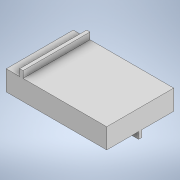
# Autodesk Inventor part: 水平滑盖
Saved by Autodesk Inventor 2020 (Build 240168000, 168)
## iProperties
Created: 2021-04-06
Part Number: 水平滑盖
Material: 常规
Document SubType Name: Modeling
Designer: 70929
Density: 1 g/cm^3
Appearance: 默认
Author: 70929
Autodesk Inventor part; units mm, degrees
ref_plane "YZ Plane" through (0, 0, 0) normal (1, 0, 0) x (0, 1, 0)
ref_plane "XZ Plane" through (0, 0, 0) normal (0, 1, 0) x (-1, 0, 0)
ref_plane "XY Plane" through (0, 0, 0) normal (0, 0, 1) x (1, 0, 0)
sketch "草图3" plane through (0, 0, 0) normal (0, 1, 0) x (-1, 0, 0)
  line L0 (-75, 50) -> (75, 50)
  line L1 (75, 50) -> (75, -50)
  line L2 (75, -50) -> (-75, -50)
  line L3 (-75, -50) -> (-75, 50)
  line L4 (-75, 50) -> (75, -50) construction
  line L5 (75, 50) -> (-75, -50) construction
  point P0 (0, 0)
  dimension "d21" = 150
  dimension "d22" = 100
  constraints: 12 end point, 2 midpoint, 2 parallel, 1 horizontal, 1 perpendicular
  measures "d21" distance of L1.end L2.end
  measures "d22" distance of L2.end L0.start
extrude "拉伸3" add sketch "草图3" against normal mid plane 30
sketch "草图4" plane through (0, 15, 0) normal (0, 1, 0) x (1, 0, 0)
  line L0 (-75, -50) -> (-55, -50)
  line L1 (75, -50) -> (-75, -50) projected
  line L2 (-55, -50) -> (-55, 50)
  line L3 (-55, 50) -> (-50, 50)
  line L4 (-75, 50) -> (75, 50) projected
  line L5 (-50, 50) -> (-50, -50)
  line L6 (-50, -50) -> (-55, -50)
  point P0 (0, 0)
  dimension "d25" = 20
  dimension "d31" = 5
  constraints: 10 end point, 3 perpendicular, 3 point on line
  measures "d25" distance of L0.start L0.end
  measures "d31" distance of L2.end L3.end
extrude "拉伸4" add sketch "草图4" along normal blind 10
sketch "草图5" plane through (0, -15, 0) normal (0, -1, 0) x (1, 0, 0)
  line L0 (75, 50) -> (75, -50) projected
  line L1 (-75, 2.5) -> (75, 2.5)
  line L2 (75, 2.5) -> (75, -2.5)
  line L3 (75, -2.5) -> (-75, -2.5)
  line L4 (-75, -2.5) -> (-75, 2.5)
  line L5 (-75, 2.5) -> (75, -2.5) construction
  line L6 (75, 2.5) -> (-75, -2.5) construction
  point P0 (0, 0)
  point P1 (75, 2.5)
  dimension "d28" = 5
  constraints: 12 end point, 2 midpoint, 2 parallel, 1 horizontal, 1 perpendicular, 1 point on line
  measures "d28" distance of L1.end L2.end
extrude "拉伸5" add sketch "草图5" along normal blind 10
